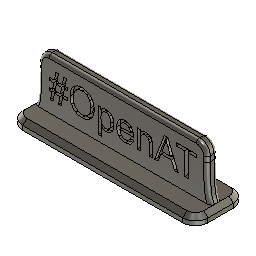
OpenAT_Placard (Autodesk Fusion 360 design; units mm, degrees)
Autodesk Fusion 360 part; units mm, degrees
sketch "Front_Sketch" plane through (0, 0, 0) normal (0, 1, 0) x (1, 0, 0)
  line L0 (-22, 0) -> (22, 0)
  line L1 (22, 0) -> (22, -2)
  line L2 (22, -2) -> (-22, -2)
  line L3 (-22, -2) -> (-22, 0)
  line L4 (-20, -2) -> (20, -2)
  line L5 (20, -2) -> (20, -14)
  line L6 (20, -14) -> (-20, -14)
  line L7 (-20, -14) -> (-20, -2)
  line L8 (0, 0) -> (0, -14) construction
  line L9 (-20, -14) -> (20, -2) construction
  line L10 (-20, -2) -> (20, -14) construction
  line L11 (-20, -2) -> (20, -2) construction
  line L12 (20, -2) -> (20, -14) construction
  line L13 (20, -14) -> (-20, -14) construction
  line L14 (-20, -14) -> (-20, -2) construction
  spline S0 degree 5 poles (-20, -14) (-20, -13.7084) (-19.9988, -13.0095) (-19.9936, -11.6148) (-19.9912, -9.2079) (-20.0681, -5.9453) (-20.279, -3.7303) (-20.5759, -2.6077) (-20.8465, -2.1535) (-21, -2) knots 0 0 0 0 0 0 0.2 0.4 0.6 0.8 1 1 1 1 1 1
  line L15 (-20, -14.75) -> (-20, -13.25)
  line L16 (-20.6464, -2.3536) -> (-21.3536, -1.6464)
  spline S1 degree 5 poles (21, -2) (20.8465, -2.1535) (20.5759, -2.6077) (20.279, -3.7303) (20.0681, -5.9453) (19.9912, -9.2079) (19.9936, -11.6148) (19.9988, -13.0095) (20, -13.7084) (20, -14) knots 0 0 0 0 0 0 0.2 0.4 0.6 0.8 1 1 1 1 1 1
  line L17 (20, -13.25) -> (20, -14.75)
  line L18 (21.3536, -1.6464) -> (20.6464, -2.3536)
  dimension "d4" = 6
  dimension "d5" = 2
  dimension "d6" = 2
  dimension "d7" = 12
  dimension "d19" = 40
  dimension "d23" = 45
  dimension "d24" = 45
  dimension "d25" = 1
  dimension "d26" = 1.5
  dimension "d27" = 1
  dimension "d28" = 1
  text T0 "#OpenAT" font "Arial" height 6 align centre middle in box 40 x 12 at (-20, -2) x (1, 0) y (0, -1) spacing 1 kerned
  constraint horizontal L0
  constraint vertical L1
  constraint horizontal L2
  constraint vertical L3
  constraint horizontal L4
  constraint vertical L5
  constraint horizontal L6
  constraint vertical L7
  constraint coincident L2 L4.start
  constraint midpoint L0 L8.start
  constraint midpoint L6 L8.end
  constraint coincident L8.start origin
  constraint perpendicular L0 L8
  constraint midpoint L10
  constraint horizontal L13
  constraint coincident L5.end
  constraint midpoint L6.end L15
  constraint coincident L14 L15.end
  constraint midpoint S0.end L16
  constraint midpoint L5.end L17
  constraint coincident L12 L17.start
  constraint equal L15 L17
  constraint midpoint S1.start L18
  constraint equal L16 L18
  constraint coincident S0.end L2
  constraint coincident S1.start L2
  constraint coincident L1.end L2.start
  measures "d5" distance of L0 L2
  measures "d6" distance of L1 L5
  measures "d7" distance of L2 L6
  measures "d19" distance of L5 L7
  measures "d23" angle of L2 L16
  measures "d24" angle of L2 L18
  measures "d25" distance of L18.start L18.end
  measures "d26" distance of L17.start L17.end
  measures "d27" distance of S0.end L3
  measures "d28" distance of S1.start L1
extrude "Extrude1" add sketch "Front_Sketch" along normal mid plane 2.49 contours L2 L7 S0 | L2 L5 S1 | L2 L4 L5 L6 L7 S0 L15 S1 L17
sketch "Base" plane through (0, 0, 0) normal (0, 0, 1) x (1, 0, 0)
  line L0 (22, -6) -> (-22, -6)
  line L1 (-22, -6) -> (-22, 6)
  line L2 (-22, 6) -> (22, 6)
  line L3 (22, 6) -> (22, -6)
  line L4 (22, -6) -> (-22, 6) construction
  line L5 (-22, -6) -> (22, 6) construction
  point P0 (22, 0)
  point P1 (22, 0)
  dimension "d10" = 12
  constraint horizontal L0
  constraint perpendicular L0 L1
  constraint parallel L0 L2
  constraint parallel L1 L3
  constraint coincident L4 origin
  constraint coincident L5 origin
  constraint coincident L3 P1
  measures "d10" distance of L0 L2
extrude "Extrude2" add sketch "Base" along normal up to surface (2 mm away)
fillet "Fillet1" radius 3 4 edges at (22, -6, 1) (22, 6, 1) (-22, -6, 1) (-22, 6, 1)
emboss "Emboss1" depth -0.8 profiles "Front_Sketch" section 1 text T0 onto face at (-6.6839, -1.245, 7.5273)
fillet "Fillet2" radius 2.5 2 edges at (20, 0, 14) (-20, 0, 14)
chamfer "Chamfer2" distance 1 angle 45 8 edges at (-22, 0, 2) (-21.1213, 5.1213, 2) (0, 6, 2) (21.1213, 5.1213, 2) (22, 0, 2) (21.1213, -5.1213, 2) (0, -6, 2) (-21.1213, -5.1213, 2)
fillet "Fillet3" radius 0.8 14 edges at (-20.1803, 1.245, 5.1787) (20, 1.245, 10.8949) (19.2678, 1.245, 13.2678) (0, 1.245, 14) (-19.2678, 1.245, 13.2678) (-20, 1.245, 10.8949) (20.1803, 1.245, 5.1787) (-20.1803, -1.245, 5.1787) (20, -1.245, 10.8949) (19.2678, -1.245, 13.2678) (0, -1.245, 14) (-19.2678, -1.245, 13.2678) (-20, -1.245, 10.8949) (20.1803, -1.245, 5.1787)
named bodies: "OpenAT_Placard"
